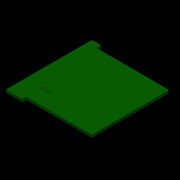
# Autodesk Inventor part: hw_DAA - PCB FPGA
Saved by Autodesk Inventor 2018 (Build 220112000, 112)
## iProperties
Created: 2024-03-13
Part Number: hw_DAA - PCB FPGA
Material: PCB
Document SubType Name: Modeling
Designer: cda1
Density: 4 g/cm^3
Appearance: PCB
Author: cda1
Autodesk Inventor part; units mm, degrees
(part 1 of 15)
ref_plane "YZ Plane" through (0, 0, 0) normal (1, 0, 0) x (0, 1, 0)
ref_plane "XZ Plane" through (0, 0, 0) normal (0, 1, 0) x (-1, 0, 0)
sketch "Boceto1" plane through (0, 0, 0) normal (0, 0, 1) x (1, 0, 0)
  line L0 (-26, 26) -> (26, 26)
  line L1 (26, 26) -> (26, -26)
  line L2 (26, -26) -> (-26, -26)
  line L3 (-26, -26) -> (-26, 26)
  line L4 (-26, 26) -> (26, -26) construction
  line L5 (26, 26) -> (-26, -26) construction
  point P0 (0, 0)
  dimension "d0" = 52
  dimension "d1" = 52
  constraints: 12 end point, 2 midpoint, 2 parallel, 1 horizontal, 1 perpendicular
  measures "d0" distance of L1.end L2.end
  measures "d1" distance of L0.end L1.end
extrude "Extrusión1" add sketch "Boceto1" against normal blind 1.742
fillet "Empalme1" radius 0.5 4 edges at (26, 26, -0.871) (-26, 26, -0.871) (-26, -26, -0.871) (26, -26, -0.871)
ref_plane "Plano de trabajo1" through (0, 0, -1.742) normal (0, 0, 1) x (1, 0, 0)
sketch "Boceto5" plane through (0, 0, 0) normal (0, 0, 1) x (1, 0, 0)
  arc A0 (25.5, -26) -> (26, -25.5) centre (25.5, -25.5) ccw construction
  line L0 (26, 25.5) -> (26, -25.5) construction
  arc A1 (26, 25.5) -> (25.5, 26) centre (25.5, 25.5) ccw construction
  line L1 (-25.5, 26) -> (25.5, 26) construction
  arc A2 (-25.5, 26) -> (-26, 25.5) centre (-25.5, 25.5) ccw construction
  line L2 (-26, -25.5) -> (-26, 25.5) construction
  arc A3 (-26, -25.5) -> (-25.5, -26) centre (-25.5, -25.5) ccw projected
  line L3 (25.5, -26) -> (-25.5, -26) projected
  line L4 (-26, -25.5) -> (-26, -28.5)
  line L5 (-26, -28.5) -> (-15.5, -28.5)
  line L6 (-15.5, -28.5) -> (-15.5, -26)
  point P0 (0, 0)
  dimension "d10" = 2.5
  dimension "d11" = 10.5
  constraints: 6 end point, 2 perpendicular, 1 point on line, 1 vertical
  measures "d10" distance of L5.end L6.end
  measures "d11" distance of L4.end L5.end
extrude "Extrusión3" add sketch "Boceto5" against normal up to surface (1.742 mm away)
sketch "Boceto6" plane through (0, 0, -1.742) normal (0, 0, -1) x (-1, 0, 0)
  arc A0 (-26, -25.5) -> (-25.5, -26) centre (-25.5, -25.5) ccw construction
  line L0 (-25.5, -26) -> (15.5, -26) construction
  line L1 (15.5, -28.5) -> (15.5, -26) construction
  line L2 (26, -28.5) -> (15.5, -28.5) construction
  line L3 (26, -28.5) -> (26, 25.5) construction
  arc A1 (26, 25.5) -> (25.5, 26) centre (25.5, 25.5) ccw construction
  line L4 (25.5, 26) -> (-25.5, 26) construction
  arc A2 (-25.5, 26) -> (-26, 25.5) centre (-25.5, 25.5) ccw construction
  line L5 (-26, 25.5) -> (-26, -25.5) construction
  line L6 (-26, 25.5) -> (-26, -25.5) construction
  line L7 (-26, 23) -> (20.107, 23)
  line L8 (20.107, 23) -> (20.107, 26)
  line L9 (20.107, 26) -> (-26, 26)
  line L10 (-26, 26) -> (-26, 23)
  point P0 (0, 0)
  dimension "d15" = 46.107
  dimension "d16" = 3
  constraints: 8 end point, 2 parallel, 2 point on line, 1 horizontal, 1 perpendicular
  measures "d15" distance of L9.end L8.end
  measures "d16" distance of L9.end L7.start
extrude "Extrusión4" cut sketch "Boceto6" against normal up to surface (1.742 mm away)
fillet "Empalme2" radius 1 1 edges at (26, 23, -0.871)
fillet "Empalme3" radius 0.5 5 edges at (-15.5, -28.5, -0.871) (-15.5, -26, -0.871) (-26, -28.5, -0.871) (-20.107, 23, -0.871) (-20.107, 26, -0.871)
sketch "Boceto17" plane through (0, 0, -1.742) normal (0, 0, -1) x (-1, 0, 0)
  circle A0 centre (16.175, -15.765) radius 0.37
  line L0 (26, -28) -> (26, 25.5) projected
  line L1 (25.5, -28.5) -> (16, -28.5) projected
  circle A1 centre (16.175, -17.035) radius 0.37
  circle A2 centre (14.905, -17.035) radius 0.37
  circle A3 centre (14.905, -15.765) radius 0.37
  circle A4 centre (13.635, -15.765) radius 0.37
  circle A5 centre (13.635, -17.035) radius 0.37
  circle A6 centre (12.365, -15.765) radius 0.37
  circle A7 centre (12.365, -17.035) radius 0.37
  circle A8 centre (11.095, -15.765) radius 0.37
  circle A9 centre (11.095, -17.035) radius 0.37
  circle A10 centre (9.825, -17.035) radius 0.37
  circle A11 centre (9.825, -15.765) radius 0.37
  point P0 (0, 0)
  dimension "d23" = 0.74
  dimension "d24" = 9.825
  dimension "d25" = 12.735
  dimension "d26" = 0.74
  dimension "d27" = 1.27
  dimension "d28" = 0.74
  dimension "d29" = 0.74
  dimension "d30" = 0.74
  dimension "d31" = 0.74
  dimension "d32" = 0.74
  dimension "d33" = 0.74
  dimension "d34" = 0.74
  dimension "d35" = 0.74
  dimension "d36" = 0.74
  dimension "d37" = 0.74
  dimension "d38" = 1.27
  dimension "d39" = 1.27
  dimension "d40" = 1.27
  dimension "d41" = 1.27
  dimension "d42" = 1.27
  constraints: 12 centre point, 10 horizontal alignment, 6 vertical alignment
  measures "d23" diameter of A0
  measures "d24" distance from line of L0 A0.centre
  measures "d25" distance from line of L1 A0.centre
  measures "d26" diameter of A1
  measures "d27" distance of A0.centre A1.centre
  measures "d28" diameter of A2
  measures "d29" diameter of A3
  measures "d30" diameter of A4
  measures "d31" diameter of A5
  measures "d32" diameter of A6
  measures "d33" diameter of A7
  measures "d34" diameter of A8
  measures "d35" diameter of A9
  measures "d36" diameter of A10
  measures "d37" diameter of A11
  measures "d38" distance of A1.centre A2.centre
  measures "d39" distance of A2.centre A5.centre
  measures "d40" distance of A5.centre A7.centre
  measures "d41" distance of A7.centre A9.centre
  measures "d42" distance of A9.centre A10.centre
extrude "Extrusión6" cut sketch "Boceto17" against normal up to surface (1.742 mm away)
sketch "TOP - 20240902" plane through (0, 0, 0) normal (0, 0, 1) x (1, 0, 0)
  arc A0 (-26, -28) -> (-25.5, -28.5) centre (-25.5, -28) ccw construction
  line L0 (-22.8, -32.942) -> (-22.8, -37.5)
  arc A1 (-22.8003, -37.5) -> (-22.7997, -37.5) centre (-22.8, -37.5) ccw
  arc A2 (-22.7997, -32.942) -> (-22.8003, -32.942) centre (-22.8, -32.942) ccw
  arc A3 (-23.3, -38) -> (-22.8, -37.5) centre (-23.3, -37.5) ccw
  arc A4 (-23.3, -37.9997) -> (-23.3, -38.0002) centre (-23.3, -38) ccw
  arc A5 (-22.7997, -37.5) -> (-22.8003, -37.5) centre (-22.8, -37.5) ccw
  line L1 (-23.3, -38) -> (-29.8, -38)
  arc A6 (-29.8, -37.9997) -> (-29.8, -38.0002) centre (-29.8, -38) ccw
  arc A7 (-23.3, -38.0002) -> (-23.3, -37.9997) centre (-23.3, -38) ccw
  arc A8 (-30.3, -37.5) -> (-29.8, -38) centre (-29.8, -37.5) ccw
  arc A9 (-30.2997, -37.5) -> (-30.3003, -37.5) centre (-30.3, -37.5) ccw
  arc A10 (-29.8, -38.0002) -> (-29.8, -37.9997) centre (-29.8, -38) ccw
  line L2 (-30.3, -37.5) -> (-30.3, -31.2)
  arc A11 (-30.2997, -31.2) -> (-30.3003, -31.2) centre (-30.3, -31.2) ccw
  arc A12 (-30.3003, -37.5) -> (-30.2997, -37.5) centre (-30.3, -37.5) ccw
  arc A13 (-30.3, -31.2) -> (-30.8, -30.7) centre (-30.8, -31.2) ccw
  arc A14 (-30.3003, -31.2) -> (-30.2997, -31.2) centre (-30.3, -31.2) ccw
  arc A15 (-30.8, -30.6998) -> (-30.8, -30.7002) centre (-30.8, -30.7) ccw
  line L3 (-30.8, -30.7) -> (-76.8, -30.7)
  arc A16 (-76.8, -30.6998) -> (-76.8, -30.7002) centre (-76.8, -30.7) ccw
  arc A17 (-30.8, -30.7002) -> (-30.8, -30.6998) centre (-30.8, -30.7) ccw
  arc A18 (-76.8, -30.7) -> (-77.3, -31.2) centre (-76.8, -31.2) ccw
  arc A19 (-76.8, -30.7002) -> (-76.8, -30.6998) centre (-76.8, -30.7) ccw
  arc A20 (-77.3003, -31.2) -> (-77.2998, -31.2) centre (-77.3001, -31.2) ccw
  line L4 (-77.3, -31.2) -> (-77.3, -49.2)
  arc A21 (-77.3003, -49.2) -> (-77.2998, -49.2) centre (-77.3001, -49.2) ccw
  arc A22 (-77.2998, -31.2) -> (-77.3003, -31.2) centre (-77.3001, -31.2) ccw
  arc A23 (-77.3, -49.2) -> (-75.3, -51.2) centre (-75.3, -49.2) ccw
  arc A24 (-77.2998, -49.2) -> (-77.3003, -49.2) centre (-77.3001, -49.2) ccw
  arc A25 (-75.3, -51.2002) -> (-75.3, -51.1998) centre (-75.3, -51.2) ccw
  line L5 (-75.3, -51.2) -> (-71.048, -51.2)
  arc A26 (-71.048, -51.2002) -> (-71.048, -51.1998) centre (-71.048, -51.2) ccw
  arc A27 (-75.3, -51.1998) -> (-75.3, -51.2002) centre (-75.3, -51.2) ccw
  arc A28 (-65.048, -57.2) -> (-71.048, -51.2) centre (-71.0482, -57.2002) ccw
  arc A29 (-65.0482, -57.2) -> (-65.0477, -57.2) centre (-65.048, -57.2) ccw
  arc A30 (-71.048, -51.1998) -> (-71.048, -51.2002) centre (-71.048, -51.2) ccw
  line L6 (-65.048, -57.2) -> (-65.048, -62.7)
  arc A31 (-65.0482, -62.7) -> (-65.0477, -62.7) centre (-65.048, -62.7) ccw
  arc A32 (-65.0477, -57.2) -> (-65.0482, -57.2) centre (-65.048, -57.2) ccw
  arc A33 (-65.048, -62.7) -> (-63.048, -64.7) centre (-63.048, -62.7) ccw
  arc A34 (-65.0477, -62.7) -> (-65.0482, -62.7) centre (-65.048, -62.7) ccw
  arc A35 (-63.048, -64.7002) -> (-63.048, -64.6997) centre (-63.048, -64.7) ccw
  line L7 (-63.048, -64.7) -> (-30.8, -64.7)
  arc A36 (-30.8, -64.7002) -> (-30.8, -64.6997) centre (-30.8, -64.7) ccw
  arc A37 (-63.048, -64.6997) -> (-63.048, -64.7002) centre (-63.048, -64.7) ccw
  arc A38 (-30.8, -64.7) -> (-30.3, -64.2) centre (-30.8, -64.2) ccw
  arc A39 (-30.8, -64.6997) -> (-30.8, -64.7002) centre (-30.8, -64.7) ccw
  arc A40 (-30.2997, -64.2) -> (-30.3003, -64.2) centre (-30.3, -64.2) ccw
  line L8 (-30.3, -64.2) -> (-30.3, -59.8)
  arc A41 (-30.2997, -59.8) -> (-30.3003, -59.8) centre (-30.3, -59.8) ccw
  arc A42 (-30.3003, -64.2) -> (-30.2997, -64.2) centre (-30.3, -64.2) ccw
  arc A43 (-29.8, -59.3) -> (-30.3, -59.8) centre (-29.8, -59.8) ccw
  arc A44 (-29.8, -59.3002) -> (-29.8, -59.2998) centre (-29.8, -59.3) ccw
  arc A45 (-30.3003, -59.8) -> (-30.2997, -59.8) centre (-30.3, -59.8) ccw
  line L9 (-29.8, -59.3) -> (-23.3, -59.3)
  arc A46 (-23.3, -59.3002) -> (-23.3, -59.2998) centre (-23.3, -59.3) ccw
  arc A47 (-29.8, -59.2998) -> (-29.8, -59.3002) centre (-29.8, -59.3) ccw
  arc A48 (-22.8, -59.8) -> (-23.3, -59.3) centre (-23.3, -59.8) ccw
  arc A49 (-22.8003, -59.8) -> (-22.7997, -59.8) centre (-22.8, -59.8) ccw
  arc A50 (-23.3, -59.2998) -> (-23.3, -59.3002) centre (-23.3, -59.3) ccw
  line L10 (-22.8, -59.8) -> (-22.8, -62.458)
  arc A51 (-22.8003, -62.458) -> (-22.7997, -62.458) centre (-22.8, -62.458) ccw
  arc A52 (-22.7997, -59.8) -> (-22.8003, -59.8) centre (-22.8, -59.8) ccw
  arc A53 (-22.8, -62.458) -> (-22.3, -62.958) centre (-22.3, -62.458) ccw
  arc A54 (-22.7997, -62.458) -> (-22.8003, -62.458) centre (-22.8, -62.458) ccw
  arc A55 (-22.3, -62.9582) -> (-22.3, -62.9577) centre (-22.3, -62.958) ccw
  line L11 (-22.3, -62.958) -> (-16, -62.958)
  arc A56 (-16, -62.9582) -> (-16, -62.9577) centre (-16, -62.958) ccw
  arc A57 (-22.3, -62.9577) -> (-22.3, -62.9582) centre (-22.3, -62.958) ccw
  arc A58 (-16, -62.958) -> (-15.5, -62.458) centre (-16, -62.458) ccw
  arc A59 (-16, -62.9577) -> (-16, -62.9582) centre (-16, -62.958) ccw
  arc A60 (-15.4998, -62.458) -> (-15.5002, -62.458) centre (-15.5, -62.458) ccw
  line L12 (-15.5, -62.458) -> (-15.5, -60.4)
  arc A61 (-15.4998, -60.4) -> (-15.5002, -60.4) centre (-15.5, -60.4) ccw
  arc A62 (-15.5002, -62.458) -> (-15.4998, -62.458) centre (-15.5, -62.458) ccw
  arc A63 (25.5, -120.6) -> (26, -120.1) centre (25.5, -120.1) ccw
  arc A64 (25.5, -120.5998) -> (25.5, -120.6003) centre (25.5, -120.6001) ccw
  arc A65 (26.0003, -120.1) -> (25.9998, -120.1) centre (26, -120.1) ccw
  line L13 (25.5, -120.6) -> (-25.5, -120.6)
  arc A66 (-25.5, -120.5998) -> (-25.5, -120.6003) centre (-25.5, -120.6001) ccw
  arc A67 (25.5, -120.6003) -> (25.5, -120.5998) centre (25.5, -120.6001) ccw
  arc A68 (-26, -120.1) -> (-25.5, -120.6) centre (-25.5, -120.1) ccw
  arc A69 (-25.9997, -120.1) -> (-26.0002, -120.1) centre (-26, -120.1) ccw
  arc A70 (-25.5, -120.6003) -> (-25.5, -120.5998) centre (-25.5, -120.6001) ccw
  line L14 (-26, -120.1) -> (-26, -66.6)
  arc A71 (-25.9997, -66.6) -> (-26.0002, -66.6) centre (-26, -66.6) ccw
  arc A72 (-26.0002, -120.1) -> (-25.9997, -120.1) centre (-26, -120.1) ccw
  arc A73 (-25.5, -66.1) -> (-26, -66.6) centre (-25.5, -66.6) ccw
  arc A74 (-25.5, -66.1003) -> (-25.5, -66.0997) centre (-25.5, -66.1) ccw
  arc A75 (-26.0002, -66.6) -> (-25.9997, -66.6) centre (-26, -66.6) ccw
  line L15 (-25.5, -66.1) -> (-16, -66.1)
  arc A76 (-16, -66.1003) -> (-16, -66.0997) centre (-16, -66.1) ccw
  arc A77 (-25.5, -66.0997) -> (-25.5, -66.1003) centre (-25.5, -66.1) ccw
  arc A78 (-15.5, -66.6) -> (-16, -66.1) centre (-16, -66.6) ccw
  arc A79 (-15.5002, -66.6) -> (-15.4998, -66.6) centre (-15.5, -66.6) ccw
  arc A80 (-16, -66.0997) -> (-16, -66.1003) centre (-16, -66.1) ccw
  line L16 (-15.5, -66.6) -> (-15.5, -72.9)
  arc A81 (-15.5002, -72.9) -> (-15.4998, -72.9) centre (-15.5, -72.9) ccw
  arc A82 (-15.4998, -66.6) -> (-15.5002, -66.6) centre (-15.5, -66.6) ccw
  arc A83 (-15.5, -72.9) -> (-15, -73.4) centre (-15, -72.9) ccw
  arc A84 (-15.4998, -72.9) -> (-15.5002, -72.9) centre (-15.5, -72.9) ccw
  arc A85 (-15, -73.4002) -> (-15, -73.3997) centre (-15, -73.4) ccw
  line L17 (-15, -59.9) -> (-13.5, -59.9)
  arc A86 (-13.5, -59.9002) -> (-13.5, -59.8998) centre (-13.5, -59.9) ccw
  arc A87 (-15, -59.8998) -> (-15, -59.9002) centre (-15, -59.9) ccw
  arc A88 (-13, -60.4) -> (-13.5, -59.9) centre (-13.5, -60.4) ccw
  arc A89 (-13.0002, -60.4) -> (-12.9998, -60.4) centre (-13, -60.4) ccw
  arc A90 (-13.5, -59.8998) -> (-13.5, -59.9002) centre (-13.5, -59.9) ccw
  line L18 (-13, -60.4) -> (-13, -72.9)
  arc A91 (-13.0002, -72.9) -> (-12.9998, -72.9) centre (-13, -72.9) ccw
  arc A92 (-12.9998, -60.4) -> (-13.0002, -60.4) centre (-13, -60.4) ccw
  arc A93 (-13.5, -73.4) -> (-13, -72.9) centre (-13.5, -72.9) ccw
  arc A94 (-13.5, -73.3997) -> (-13.5, -73.4002) centre (-13.5, -73.4) ccw
  arc A95 (-12.9998, -72.9) -> (-13.0002, -72.9) centre (-13, -72.9) ccw
  line L19 (-13.5, -73.4) -> (-15, -73.4)
  arc A96 (-15, -73.3997) -> (-15, -73.4002) centre (-15, -73.4) ccw
  arc A97 (-13.5, -73.4002) -> (-13.5, -73.3997) centre (-13.5, -73.4) ccw
  arc A98 (26, -73.9) -> (25.5, -73.4) centre (25.5, -73.9) ccw
  arc A99 (25.9998, -73.9) -> (26.0003, -73.9) centre (26, -73.9) ccw
  arc A100 (25.5, -73.3997) -> (25.5, -73.4002) centre (25.5, -73.4) ccw
  line L20 (26, -73.9) -> (26, -120.1)
  arc A101 (25.9998, -120.1) -> (26.0003, -120.1) centre (26, -120.1) ccw
  arc A102 (26.0003, -73.9) -> (25.9998, -73.9) centre (26, -73.9) ccw
  line L21 (7.4, 23.5) -> (7.4, 31.9)
  arc A103 (7.4002, 31.9) -> (7.3998, 31.9) centre (7.4, 31.9) ccw
  arc A104 (7.3998, 23.5) -> (7.4002, 23.5) centre (7.4, 23.5) ccw
  arc A105 (7.9, 32.4) -> (7.4, 31.9) centre (7.9, 31.9) ccw
  arc A106 (7.9, 32.3998) -> (7.9, 32.4002) centre (7.9, 32.4) ccw
  arc A107 (7.3998, 31.9) -> (7.4002, 31.9) centre (7.4, 31.9) ccw
  line L22 (7.9, 32.4) -> (12.55, 32.4)
  arc A108 (12.55, 32.3998) -> (12.55, 32.4002) centre (12.55, 32.4) ccw
  arc A109 (7.9, 32.4002) -> (7.9, 32.3998) centre (7.9, 32.4) ccw
  arc A110 (7.4, 23.5) -> (7.9, 23) centre (7.9, 23.5) ccw
  arc A111 (7.4002, 23.5) -> (7.3998, 23.5) centre (7.4, 23.5) ccw
  arc A112 (7.9, 22.9998) -> (7.9, 23.0002) centre (7.9, 23) ccw
  line L23 (7.9, 23) -> (25, 23)
  arc A113 (25, 22.9998) -> (25, 23.0002) centre (25, 23) ccw
  arc A114 (7.9, 23.0002) -> (7.9, 22.9998) centre (7.9, 23) ccw
  arc A115 (12.55, 32.4) -> (13.05, 32.9) centre (12.55, 32.9) ccw
  arc A116 (12.55, 32.4002) -> (12.55, 32.3998) centre (12.55, 32.4) ccw
  arc A117 (13.0503, 32.9) -> (13.0498, 32.9) centre (13.05, 32.9) ccw
  line L24 (13.05, 32.9) -> (13.05, 40.1)
  arc A118 (13.0503, 40.1) -> (13.0498, 40.1) centre (13.05, 40.1) ccw
  arc A119 (13.0498, 32.9) -> (13.0503, 32.9) centre (13.05, 32.9) ccw
  arc A120 (13.55, 40.6) -> (13.05, 40.1) centre (13.55, 40.1) ccw
  arc A121 (13.55, 40.5998) -> (13.55, 40.6003) centre (13.55, 40.6) ccw
  arc A122 (13.0498, 40.1) -> (13.0503, 40.1) centre (13.05, 40.1) ccw
  line L25 (13.55, 40.6) -> (36.8, 40.6)
  arc A123 (36.8, 40.5998) -> (36.8, 40.6003) centre (36.8, 40.6) ccw
  arc A124 (13.55, 40.6003) -> (13.55, 40.5998) centre (13.55, 40.6) ccw
  arc A125 (37.3, 40.1) -> (36.8, 40.6) centre (36.8, 40.1) ccw
  arc A126 (37.2998, 40.1) -> (37.3003, 40.1) centre (37.3, 40.1) ccw
  arc A127 (36.8, 40.6003) -> (36.8, 40.5998) centre (36.8, 40.6) ccw
  line L26 (37.3, 40.1) -> (37.3, 36)
  arc A128 (37.2998, 36) -> (37.3003, 36) centre (37.3, 36) ccw
  arc A129 (37.3003, 40.1) -> (37.2998, 40.1) centre (37.3, 40.1) ccw
  arc A130 (36.8, 35.5) -> (37.3, 36) centre (36.8, 36) ccw
  arc A131 (36.8, 35.5002) -> (36.8, 35.4998) centre (36.8, 35.5) ccw
  arc A132 (37.3003, 36) -> (37.2998, 36) centre (37.3, 36) ccw
  line L27 (36.8, 35.5) -> (34.4, 35.5)
  arc A133 (34.4, 35.5002) -> (34.4, 35.4998) centre (34.4, 35.5) ccw
  arc A134 (36.8, 35.4998) -> (36.8, 35.5002) centre (36.8, 35.5) ccw
  arc A135 (34.4, 35.5) -> (33.9, 35) centre (34.4, 35) ccw
  arc A136 (34.4, 35.4998) -> (34.4, 35.5002) centre (34.4, 35.5) ccw
  arc A137 (33.8998, 35) -> (33.9002, 35) centre (33.9, 35) ccw
  line L28 (33.9, 35) -> (33.9, 30.9)
  arc A138 (33.8998, 30.9) -> (33.9002, 30.9) centre (33.9, 30.9) ccw
  arc A139 (33.9002, 35) -> (33.8998, 35) centre (33.9, 35) ccw
  arc A140 (33.9, 30.9) -> (34.4, 30.4) centre (34.4, 30.9) ccw
  arc A141 (33.9002, 30.9) -> (33.8998, 30.9) centre (33.9, 30.9) ccw
  arc A142 (34.4, 30.3998) -> (34.4, 30.4002) centre (34.4, 30.4) ccw
  line L29 (38.9, 31.8) -> (38.9, 30.9)
  arc A143 (38.8998, 30.9) -> (38.9002, 30.9) centre (38.9, 30.9) ccw
  arc A144 (38.9002, 31.8) -> (38.8998, 31.8) centre (38.9, 31.8) ccw
  arc A145 (38.4, 30.4) -> (38.9, 30.9) centre (38.4, 30.9) ccw
  arc A146 (38.4, 30.4002) -> (38.4, 30.3998) centre (38.4, 30.4) ccw
  arc A147 (38.9002, 30.9) -> (38.8998, 30.9) centre (38.9, 30.9) ccw
  line L30 (38.4, 30.4) -> (34.4, 30.4)
  arc A148 (34.4, 30.4002) -> (34.4, 30.3998) centre (34.4, 30.4) ccw
  arc A149 (38.4, 30.3998) -> (38.4, 30.4002) centre (38.4, 30.4) ccw
  line L31 (77.3, 32.8) -> (77.3, 50.2)
  arc A150 (77.3002, 50.2) -> (77.2998, 50.2) centre (77.3, 50.2) ccw
  arc A151 (77.2998, 32.8) -> (77.3002, 32.8) centre (77.3, 32.8) ccw
  arc A152 (77.8, 50.7) -> (77.3, 50.2) centre (77.8, 50.2) ccw
  arc A153 (77.8, 50.6998) -> (77.8, 50.7003) centre (77.8, 50.7) ccw
  arc A154 (77.2998, 50.2) -> (77.3002, 50.2) centre (77.3, 50.2) ccw
  line L32 (77.8, 50.7) -> (79.8, 50.7)
  arc A155 (79.8, 50.6998) -> (79.8, 50.7003) centre (79.8, 50.7) ccw
  arc A156 (77.8, 50.7003) -> (77.8, 50.6998) centre (77.8, 50.7) ccw
  arc A157 (79.8, 50.7) -> (80.3, 51.2) centre (79.8, 51.2) ccw
  arc A158 (79.8, 50.7003) -> (79.8, 50.6998) centre (79.8, 50.7) ccw
  arc A159 (80.3002, 51.2) -> (80.2998, 51.2) centre (80.3, 51.2) ccw
  line L33 (80.3, 51.2) -> (80.3, 56.4)
  arc A160 (80.3002, 56.4) -> (80.2998, 56.4) centre (80.3, 56.4) ccw
  arc A161 (80.2998, 51.2) -> (80.3002, 51.2) centre (80.3, 51.2) ccw
  arc A162 (80.3, 56.4) -> (79.8, 56.9) centre (79.8, 56.4) ccw
  arc A163 (80.2998, 56.4) -> (80.3002, 56.4) centre (80.3, 56.4) ccw
  arc A164 (79.8, 56.9002) -> (79.8, 56.8998) centre (79.8, 56.9) ccw
  line L34 (79.8, 56.9) -> (58.9, 56.9)
  arc A165 (58.9, 56.9002) -> (58.9, 56.8998) centre (58.9, 56.9) ccw
  arc A166 (79.8, 56.8998) -> (79.8, 56.9002) centre (79.8, 56.9) ccw
  line L35 (54.4, 31.3) -> (57.9, 31.3)
  arc A167 (57.9, 31.2998) -> (57.9, 31.3002) centre (57.9, 31.3) ccw
  arc A168 (54.4, 31.3002) -> (54.4, 31.2998) centre (54.4, 31.3) ccw
  arc A169 (57.9, 31.3) -> (58.4, 31.8) centre (57.9, 31.8) ccw
  arc A170 (57.9, 31.3002) -> (57.9, 31.2998) centre (57.9, 31.3) ccw
  arc A171 (58.4003, 31.8) -> (58.3998, 31.8) centre (58.4, 31.8) ccw
  arc A172 (58.9, 32.3) -> (58.4, 31.8) centre (58.9, 31.8) ccw
  arc A173 (58.9, 32.2998) -> (58.9, 32.3002) centre (58.9, 32.3) ccw
  arc A174 (58.3998, 31.8) -> (58.4003, 31.8) centre (58.4, 31.8) ccw
  line L36 (58.9, 32.3) -> (76.8, 32.3)
  arc A175 (76.8, 32.2998) -> (76.8, 32.3002) centre (76.8, 32.3) ccw
  arc A176 (58.9, 32.3002) -> (58.9, 32.2998) centre (58.9, 32.3) ccw
  arc A177 (76.8, 32.3) -> (77.3, 32.8) centre (76.8, 32.8) ccw
  arc A178 (76.8, 32.3002) -> (76.8, 32.2998) centre (76.8, 32.3) ccw
  arc A179 (77.3002, 32.8) -> (77.2998, 32.8) centre (77.3, 32.8) ccw
  arc A180 (53.9, 31.8) -> (54.4, 31.3) centre (54.4, 31.8) ccw
  arc A181 (53.9003, 31.8) -> (53.8998, 31.8) centre (53.9, 31.8) ccw
  arc A182 (54.4, 31.2998) -> (54.4, 31.3002) centre (54.4, 31.3) ccw
  arc A183 (53.9, 31.8) -> (53.4, 32.3) centre (53.4, 31.8) ccw
  arc A184 (53.8998, 31.8) -> (53.9003, 31.8) centre (53.9, 31.8) ccw
  arc A185 (53.4, 32.3002) -> (53.4, 32.2998) centre (53.4, 32.3) ccw
  line L37 (53.4, 32.3) -> (39.4, 32.3)
  arc A186 (39.4, 32.3002) -> (39.4, 32.2998) centre (39.4, 32.3) ccw
  arc A187 (53.4, 32.2998) -> (53.4, 32.3002) centre (53.4, 32.3) ccw
  arc A188 (39.4, 32.3) -> (38.9, 31.8) centre (39.4, 31.8) ccw
  arc A189 (39.4, 32.2998) -> (39.4, 32.3002) centre (39.4, 32.3) ccw
  arc A190 (38.8998, 31.8) -> (38.9002, 31.8) centre (38.9, 31.8) ccw
  line L38 (36.8, 52) -> (13.55, 52)
  arc A191 (13.55, 52.0003) -> (13.55, 51.9998) centre (13.55, 52) ccw
  arc A192 (36.8, 51.9998) -> (36.8, 52.0003) centre (36.8, 52) ccw
  arc A193 (13.05, 52.5) -> (13.55, 52) centre (13.55, 52.5) ccw
  arc A194 (13.0503, 52.5) -> (13.0498, 52.5) centre (13.05, 52.5) ccw
  arc A195 (13.55, 51.9998) -> (13.55, 52.0003) centre (13.55, 52) ccw
  line L39 (13.05, 52.5) -> (13.05, 59.358)
  arc A196 (13.0503, 59.358) -> (13.0498, 59.358) centre (13.05, 59.358) ccw
  arc A197 (13.0498, 52.5) -> (13.0503, 52.5) centre (13.05, 52.5) ccw
  arc A198 (13.05, 59.358) -> (12.55, 59.858) centre (12.55, 59.358) ccw
  arc A199 (13.0498, 59.358) -> (13.0503, 59.358) centre (13.05, 59.358) ccw
  arc A200 (12.55, 59.8582) -> (12.55, 59.8578) centre (12.55, 59.858) ccw
  line L40 (12.55, 59.858) -> (-27.242, 59.858)
  arc A201 (-27.242, 59.8582) -> (-27.242, 59.8578) centre (-27.242, 59.858) ccw
  arc A202 (12.55, 59.8578) -> (12.55, 59.8582) centre (12.55, 59.858) ccw
  arc A203 (36.8, 52) -> (37.3, 52.5) centre (36.8, 52.5) ccw
  arc A204 (36.8, 52.0003) -> (36.8, 51.9998) centre (36.8, 52) ccw
  arc A205 (37.3003, 52.5) -> (37.2998, 52.5) centre (37.3, 52.5) ccw
  line L41 (37.3, 52.5) -> (37.3, 53.2)
  arc A206 (37.3003, 53.2) -> (37.2998, 53.2) centre (37.3, 53.2) ccw
  arc A207 (37.2998, 52.5) -> (37.3003, 52.5) centre (37.3, 52.5) ccw
  arc A208 (-27.242, 59.858) -> (-27.742, 59.358) centre (-27.242, 59.358) ccw
  arc A209 (-27.242, 59.8578) -> (-27.242, 59.8582) centre (-27.242, 59.858) ccw
  arc A210 (-27.7423, 59.358) -> (-27.7417, 59.358) centre (-27.742, 59.358) ccw
  line L42 (-27.742, 59.358) -> (-27.742, 29.842)
  arc A211 (-27.7423, 29.842) -> (-27.7417, 29.842) centre (-27.742, 29.842) ccw
  arc A212 (-27.7417, 59.358) -> (-27.7423, 59.358) centre (-27.742, 59.358) ccw
  arc A213 (37.3, 53.2) -> (36.8, 53.7) centre (36.8, 53.2) ccw
  arc A214 (37.2998, 53.2) -> (37.3003, 53.2) centre (37.3, 53.2) ccw
  arc A215 (36.8, 53.7003) -> (36.8, 53.6998) centre (36.8, 53.7) ccw
  line L43 (36.8, 53.7) -> (34.4, 53.7)
  arc A216 (34.4, 53.7003) -> (34.4, 53.6998) centre (34.4, 53.7) ccw
  arc A217 (36.8, 53.6998) -> (36.8, 53.7003) centre (36.8, 53.7) ccw
  arc A218 (33.9, 54.2) -> (34.4, 53.7) centre (34.4, 54.2) ccw
  arc A219 (33.9002, 54.2) -> (33.8998, 54.2) centre (33.9, 54.2) ccw
  arc A220 (34.4, 53.6998) -> (34.4, 53.7003) centre (34.4, 53.7) ccw
  line L44 (33.9, 54.2) -> (33.9, 58.3)
  arc A221 (33.9002, 58.3) -> (33.8998, 58.3) centre (33.9, 58.3) ccw
  arc A222 (33.8998, 54.2) -> (33.9002, 54.2) centre (33.9, 54.2) ccw
  line L45 (-15, -26) -> (-13.5, -26)
  arc A223 (-13.5, -26.0002) -> (-13.5, -25.9997) centre (-13.5, -26) ccw
  arc A224 (-15, -25.9997) -> (-15, -26.0002) centre (-15, -26) ccw
  arc A225 (-13, -26.5) -> (-13.5, -26) centre (-13.5, -26.5) ccw
  arc A226 (-13.0002, -26.5) -> (-12.9998, -26.5) centre (-13, -26.5) ccw
  arc A227 (-13.5, -25.9997) -> (-13.5, -26.0002) centre (-13.5, -26) ccw
  line L46 (-13, -26.5) -> (-13, -35)
  arc A228 (-13.0002, -35) -> (-12.9998, -35) centre (-13, -35) ccw
  arc A229 (-12.9998, -26.5) -> (-13.0002, -26.5) centre (-13, -26.5) ccw
  arc A230 (-13.5, -35.5) -> (-13, -35) centre (-13.5, -35) ccw
  arc A231 (-13.5, -35.4997) -> (-13.5, -35.5002) centre (-13.5, -35.5) ccw
  arc A232 (-12.9998, -35) -> (-13.0002, -35) centre (-13, -35) ccw
  line L47 (-13.5, -35.5) -> (-15, -35.5)
  arc A233 (-15, -35.4997) -> (-15, -35.5002) centre (-15, -35.5) ccw
  arc A234 (-13.5, -35.5002) -> (-13.5, -35.4997) centre (-13.5, -35.5) ccw
  arc A235 (-15, -26) -> (-15.5, -26.5) centre (-15, -26.5) ccw
  arc A236 (-15, -26.0002) -> (-15, -25.9997) centre (-15, -26) ccw
  arc A237 (-15.5002, -26.5) -> (-15.4998, -26.5) centre (-15.5, -26.5) ccw
  line L48 (-15.5, -26.5) -> (-15.5, -28)
  arc A238 (-15.5002, -28) -> (-15.4998, -28) centre (-15.5, -28) ccw
  arc A239 (-15.4998, -26.5) -> (-15.5002, -26.5) centre (-15.5, -26.5) ccw
  arc A240 (-16, -28.5) -> (-15.5, -28) centre (-16, -28) ccw
  arc A241 (-16, -28.4997) -> (-16, -28.5002) centre (-16, -28.5) ccw
  arc A242 (-15.4998, -28) -> (-15.5002, -28) centre (-15.5, -28) ccw
  line L49 (-16, -28.5) -> (-25.5, -28.5)
  arc A243 (-25.5, -28.4997) -> (-25.5, -28.5002) centre (-25.5, -28.5) ccw
  arc A244 (-16, -28.5002) -> (-16, -28.4997) centre (-16, -28.5) ccw
  arc A245 (-26, -28) -> (-25.5, -28.5) centre (-25.5, -28) ccw
  arc A246 (-25.9997, -28) -> (-26.0002, -28) centre (-26, -28) ccw
  arc A247 (-25.5, -28.5002) -> (-25.5, -28.4997) centre (-25.5, -28.5) ccw
  line L50 (-26, -28) -> (-26, 25.5)
  arc A248 (-25.9997, 25.5) -> (-26.0002, 25.5) centre (-26, 25.5) ccw
  arc A249 (-26.0002, -28) -> (-25.9997, -28) centre (-26, -28) ccw
  arc A250 (-25.5, 26) -> (-26, 25.5) centre (-25.5, 25.5) ccw
  arc A251 (-25.5, 25.9998) -> (-25.5, 26.0002) centre (-25.5, 26) ccw
  arc A252 (-26.0002, 25.5) -> (-25.9997, 25.5) centre (-26, 25.5) ccw
  line L51 (-25.5, 26) -> (-20.6, 26)
  arc A253 (-20.6, 25.9998) -> (-20.6, 26.0002) centre (-20.6, 26) ccw
  arc A254 (-25.5, 26.0002) -> (-25.5, 25.9998) centre (-25.5, 26) ccw
  arc A255 (-20.1, 25.5) -> (-20.6, 26) centre (-20.6, 25.5) ccw
  arc A256 (-20.1002, 25.5) -> (-20.0998, 25.5) centre (-20.1, 25.5) ccw
  arc A257 (-20.6, 26.0002) -> (-20.6, 25.9998) centre (-20.6, 26) ccw
  line L52 (-20.1, 25.5) -> (-20.1, 23.5)
  arc A258 (-20.1002, 23.5) -> (-20.0998, 23.5) centre (-20.1, 23.5) ccw
  arc A259 (-20.0998, 25.5) -> (-20.1002, 25.5) centre (-20.1, 25.5) ccw
  arc A260 (-20.1, 23.5) -> (-19.6, 23) centre (-19.6, 23.5) ccw
  arc A261 (-20.0998, 23.5) -> (-20.1002, 23.5) centre (-20.1, 23.5) ccw
  arc A262 (-19.6, 22.9998) -> (-19.6, 23.0002) centre (-19.6, 23) ccw
  line L53 (-19.6, 32.4) -> (-18.3, 32.4)
  arc A263 (-18.3, 32.3998) -> (-18.3, 32.4002) centre (-18.3, 32.4) ccw
  arc A264 (-19.6, 32.4002) -> (-19.6, 32.3998) centre (-19.6, 32.4) ccw
  arc A265 (-17.8, 31.9) -> (-18.3, 32.4) centre (-18.3, 31.9) ccw
  arc A266 (-17.8002, 31.9) -> (-17.7998, 31.9) centre (-17.8, 31.9) ccw
  arc A267 (-18.3, 32.4002) -> (-18.3, 32.3998) centre (-18.3, 32.4) ccw
  line L54 (-17.8, 31.9) -> (-17.8, 23.5)
  arc A268 (-17.8002, 23.5) -> (-17.7998, 23.5) centre (-17.8, 23.5) ccw
  arc A269 (-17.7998, 31.9) -> (-17.8002, 31.9) centre (-17.8, 31.9) ccw
  arc A270 (-18.3, 23) -> (-17.8, 23.5) centre (-18.3, 23.5) ccw
  arc A271 (-18.3, 23.0002) -> (-18.3, 22.9998) centre (-18.3, 23) ccw
  arc A272 (-17.7998, 23.5) -> (-17.8002, 23.5) centre (-17.8, 23.5) ccw
  line L55 (-18.3, 23) -> (-19.6, 23)
  arc A273 (-19.6, 23.0002) -> (-19.6, 22.9998) centre (-19.6, 23) ccw
  arc A274 (-18.3, 22.9998) -> (-18.3, 23.0002) centre (-18.3, 23) ccw
  arc A275 (26, 22) -> (25, 23) centre (25, 22) ccw
  arc A276 (25.9998, 22) -> (26.0003, 22) centre (26, 22) ccw
  arc A277 (25, 23.0002) -> (25, 22.9998) centre (25, 23) ccw
  line L56 (26, 22) -> (26, -25.5)
  arc A278 (25.9998, -25.5) -> (26.0003, -25.5) centre (26, -25.5) ccw
  arc A279 (26.0003, 22) -> (25.9998, 22) centre (26, 22) ccw
  arc A280 (25.5, -26) -> (26, -25.5) centre (25.5, -25.5) ccw
  arc A281 (25.5, -25.9997) -> (25.5, -26.0002) centre (25.5, -26) ccw
  arc A282 (26.0003, -25.5) -> (25.9998, -25.5) centre (26, -25.5) ccw
  line L57 (-15.5, -35) -> (-15.5, -32.942)
  arc A283 (-15.4998, -32.942) -> (-15.5002, -32.942) centre (-15.5, -32.942) ccw
  arc A284 (-15.5002, -35) -> (-15.4998, -35) centre (-15.5, -35) ccw
  arc A285 (-15.5, -32.942) -> (-16, -32.442) centre (-16, -32.942) ccw
  arc A286 (-15.5002, -32.942) -> (-15.4998, -32.942) centre (-15.5, -32.942) ccw
  arc A287 (-16, -32.4418) -> (-16, -32.4422) centre (-16, -32.442) ccw
  line L58 (-16, -32.442) -> (-22.3, -32.442)
  arc A288 (-22.3, -32.4418) -> (-22.3, -32.4422) centre (-22.3, -32.442) ccw
  arc A289 (-16, -32.4422) -> (-16, -32.4418) centre (-16, -32.442) ccw
  arc A290 (-22.3, -32.442) -> (-22.8, -32.942) centre (-22.3, -32.942) ccw
  arc A291 (-22.3, -32.4422) -> (-22.3, -32.4418) centre (-22.3, -32.442) ccw
  arc A292 (-22.8003, -32.942) -> (-22.7997, -32.942) centre (-22.8, -32.942) ccw
  arc A293 (-15, -59.9) -> (-15.5, -60.4) centre (-15, -60.4) ccw
  arc A294 (-15, -59.9002) -> (-15, -59.8998) centre (-15, -59.9) ccw
  arc A295 (-15.5002, -60.4) -> (-15.4998, -60.4) centre (-15.5, -60.4) ccw
  arc A296 (25.5, -59.9) -> (26, -59.4) centre (25.5, -59.4) ccw
  arc A297 (25.5, -59.8998) -> (25.5, -59.9002) centre (25.5, -59.9) ccw
  arc A298 (26.0003, -59.4) -> (25.9998, -59.4) centre (26, -59.4) ccw
  line L59 (26, -59.4) -> (26, -36)
  arc A299 (26.0003, -36) -> (25.9998, -36) centre (26, -36) ccw
  arc A300 (25.9998, -59.4) -> (26.0003, -59.4) centre (26, -59.4) ccw
  arc A301 (26, -36) -> (25.5, -35.5) centre (25.5, -36) ccw
  arc A302 (25.9998, -36) -> (26.0003, -36) centre (26, -36) ccw
  arc A303 (25.5, -35.4997) -> (25.5, -35.5002) centre (25.5, -35.5) ccw
  arc A304 (-15.5, -35) -> (-15, -35.5) centre (-15, -35) ccw
  arc A305 (-15.4998, -35) -> (-15.5002, -35) centre (-15.5, -35) ccw
  arc A306 (-15, -35.5002) -> (-15, -35.4997) centre (-15, -35.5) ccw
  line L60 (25.5, -73.4) -> (25, -73.4)
  arc A307 (25, -73.3997) -> (25, -73.4002) centre (25, -73.4) ccw
  arc A308 (25.5, -73.4002) -> (25.5, -73.3997) centre (25.5, -73.4) ccw
  arc A309 (24.5, -72.9) -> (25, -73.4) centre (25, -72.9) ccw
  arc A310 (24.5003, -72.9) -> (24.4998, -72.9) centre (24.5, -72.9) ccw
  arc A311 (25, -73.4002) -> (25, -73.3997) centre (25, -73.4) ccw
  line L61 (24.5, -72.9) -> (24.5, -60.4)
  arc A312 (24.5003, -60.4) -> (24.4998, -60.4) centre (24.5, -60.4) ccw
  arc A313 (24.4998, -72.9) -> (24.5003, -72.9) centre (24.5, -72.9) ccw
  arc A314 (25, -59.9) -> (24.5, -60.4) centre (25, -60.4) ccw
  arc A315 (25, -59.9002) -> (25, -59.8998) centre (25, -59.9) ccw
  arc A316 (24.4998, -60.4) -> (24.5003, -60.4) centre (24.5, -60.4) ccw
  line L62 (25, -59.9) -> (25.5, -59.9)
  arc A317 (25.5, -59.9002) -> (25.5, -59.8998) centre (25.5, -59.9) ccw
  arc A318 (25, -59.8998) -> (25, -59.9002) centre (25, -59.9) ccw
  line L63 (24.5, -35) -> (24.5, -26.5)
  arc A319 (24.5003, -26.5) -> (24.4998, -26.5) centre (24.5, -26.5) ccw
  arc A320 (24.4998, -35) -> (24.5003, -35) centre (24.5, -35) ccw
  arc A321 (25, -26) -> (24.5, -26.5) centre (25, -26.5) ccw
  arc A322 (25, -26.0002) -> (25, -25.9997) centre (25, -26) ccw
  arc A323 (24.4998, -26.5) -> (24.5003, -26.5) centre (24.5, -26.5) ccw
  line L64 (25, -26) -> (25.5, -26)
  arc A324 (25.5, -26.0002) -> (25.5, -25.9997) centre (25.5, -26) ccw
  arc A325 (25, -25.9997) -> (25, -26.0002) centre (25, -26) ccw
  arc A326 (24.5, -35) -> (25, -35.5) centre (25, -35) ccw
  arc A327 (24.5003, -35) -> (24.4998, -35) centre (24.5, -35) ccw
  arc A328 (25, -35.5002) -> (25, -35.4997) centre (25, -35.5) ccw
  line L65 (25, -35.5) -> (25.5, -35.5)
  arc A329 (25.5, -35.5002) -> (25.5, -35.4997) centre (25.5, -35.5) ccw
  arc A330 (25, -35.4997) -> (25, -35.5002) centre (25, -35.5) ccw
  arc A331 (-27.742, 29.842) -> (-27.242, 29.342) centre (-27.242, 29.842) ccw
  arc A332 (-27.7417, 29.842) -> (-27.7423, 29.842) centre (-27.742, 29.842) ccw
  arc A333 (-27.242, 29.3418) -> (-27.242, 29.3423) centre (-27.242, 29.342) ccw
  line L66 (-27.242, 29.342) -> (-20.6, 29.342)
  arc A334 (-20.6, 29.3418) -> (-20.6, 29.3423) centre (-20.6, 29.342) ccw
  arc A335 (-27.242, 29.3423) -> (-27.242, 29.3418) centre (-27.242, 29.342) ccw
  arc A336 (-20.6, 29.342) -> (-20.1, 29.842) centre (-20.6, 29.842) ccw
  arc A337 (-20.6, 29.3423) -> (-20.6, 29.3418) centre (-20.6, 29.342) ccw
  arc A338 (-20.0998, 29.842) -> (-20.1002, 29.842) centre (-20.1, 29.842) ccw
  line L67 (-20.1, 29.842) -> (-20.1, 31.9)
  arc A339 (-20.0998, 31.9) -> (-20.1002, 31.9) centre (-20.1, 31.9) ccw
  arc A340 (-20.1002, 29.842) -> (-20.0998, 29.842) centre (-20.1, 29.842) ccw
  arc A341 (-19.6, 32.4) -> (-20.1, 31.9) centre (-19.6, 31.9) ccw
  arc A342 (-19.6, 32.3998) -> (-19.6, 32.4002) centre (-19.6, 32.4) ccw
  arc A343 (-20.1002, 31.9) -> (-20.0998, 31.9) centre (-20.1, 31.9) ccw
  arc A344 (34.4, 58.8) -> (33.9, 58.3) centre (34.4, 58.3) ccw
  arc A345 (34.4, 58.7998) -> (34.4, 58.8002) centre (34.4, 58.8) ccw
  arc A346 (33.8998, 58.3) -> (33.9002, 58.3) centre (33.9, 58.3) ccw
  arc A347 (58.4, 57.4) -> (58.9, 56.9) centre (58.9, 57.4) ccw
  arc A348 (58.4003, 57.4) -> (58.3998, 57.4) centre (58.4, 57.4) ccw
  arc A349 (58.9, 56.8998) -> (58.9, 56.9002) centre (58.9, 56.9) ccw
  arc A350 (58.4, 57.4) -> (57.9, 57.9) centre (57.9, 57.4) ccw
  arc A351 (58.3998, 57.4) -> (58.4003, 57.4) centre (58.4, 57.4) ccw
  arc A352 (57.9, 57.9002) -> (57.9, 57.8998) centre (57.9, 57.9) ccw
  line L68 (57.9, 57.9) -> (54.4, 57.9)
  arc A353 (54.4, 57.9002) -> (54.4, 57.8998) centre (54.4, 57.9) ccw
  arc A354 (57.9, 57.8998) -> (57.9, 57.9002) centre (57.9, 57.9) ccw
  arc A355 (54.4, 57.9) -> (53.9, 57.4) centre (54.4, 57.4) ccw
  arc A356 (54.4, 57.8998) -> (54.4, 57.9002) centre (54.4, 57.9) ccw
  arc A357 (53.8998, 57.4) -> (53.9003, 57.4) centre (53.9, 57.4) ccw
  arc A358 (53.4, 56.9) -> (53.9, 57.4) centre (53.4, 57.4) ccw
  arc A359 (53.4, 56.9002) -> (53.4, 56.8998) centre (53.4, 56.9) ccw
  arc A360 (53.9003, 57.4) -> (53.8998, 57.4) centre (53.9, 57.4) ccw
  line L69 (53.4, 56.9) -> (39.4, 56.9)
  arc A361 (39.4, 56.9002) -> (39.4, 56.8998) centre (39.4, 56.9) ccw
  arc A362 (53.4, 56.8998) -> (53.4, 56.9002) centre (53.4, 56.9) ccw
  arc A363 (38.9, 57.4) -> (39.4, 56.9) centre (39.4, 57.4) ccw
  arc A364 (38.9002, 57.4) -> (38.8998, 57.4) centre (38.9, 57.4) ccw
  arc A365 (39.4, 56.8998) -> (39.4, 56.9002) centre (39.4, 56.9) ccw
  line L70 (38.9, 57.4) -> (38.9, 58.3)
  arc A366 (38.9002, 58.3) -> (38.8998, 58.3) centre (38.9, 58.3) ccw
  arc A367 (38.8998, 57.4) -> (38.9002, 57.4) centre (38.9, 57.4) ccw
  arc A368 (38.9, 58.3) -> (38.4, 58.8) centre (38.4, 58.3) ccw
  arc A369 (38.8998, 58.3) -> (38.9002, 58.3) centre (38.9, 58.3) ccw
  arc A370 (38.4, 58.8002) -> (38.4, 58.7998) centre (38.4, 58.8) ccw
  line L71 (38.4, 58.8) -> (34.4, 58.8)
  arc A371 (34.4, 58.8002) -> (34.4, 58.7998) centre (34.4, 58.8) ccw
  arc A372 (38.4, 58.7998) -> (38.4, 58.8002) centre (38.4, 58.8) ccw
  circle A373 centre (-36.6, -61.378) radius 2
  circle A374 centre (-36.6, -34.022) radius 2
  circle A375 centre (-19.1, -36.062) radius 2
  circle A376 centre (-23.092, 32.962) radius 2
  circle A377 centre (-9.192, 56.238) radius 2
  circle A378 centre (36.4, 56.256) radius 2
  circle A379 centre (78.021, 53.178) radius 2
  circle A380 centre (36.4, 32.98) radius 2
  circle A381 centre (56.15, 55.6) radius 2
  circle A382 centre (56.15, 33.6) radius 2
  circle A383 centre (-19.1, -59.338) radius 2
  circle A384 centre (-67.2, -34.022) radius 2
  circle A385 centre (23.035, -103.86) radius 0.37
  circle A386 centre (-13.635, -15.765) radius 0.37
  circle A387 centre (22.735, -52.24) radius 0.37
  circle A388 centre (-11.095, -17.035) radius 0.37
  circle A389 centre (44.6, 53.6) radius 1.5
  circle A390 centre (-9.825, -15.765) radius 0.37
  circle A391 centre (21.765, -107.67) radius 0.37
  circle A392 centre (21.765, -103.86) radius 0.37
  circle A393 centre (-16.175, -15.765) radius 0.37
  circle A394 centre (22.735, -47.16) radius 0.37
  circle A395 centre (21.765, -108.94) radius 0.37
  circle A396 centre (-14.905, -17.035) radius 0.37
  circle A397 centre (23.035, -106.4) radius 0.37
  circle A398 centre (21.465, -48.43) radius 0.37
  circle A399 centre (22.735, -49.7) radius 0.37
  circle A400 centre (23.035, -105.13) radius 0.37
  circle A401 centre (21.465, -50.97) radius 0.37
  circle A402 centre (44.6, 35.6) radius 1.5
  circle A403 centre (21.465, -52.24) radius 0.37
  circle A404 centre (21.765, -106.4) radius 0.37
  circle A405 centre (23.035, -108.94) radius 0.37
  circle A406 centre (-16.175, -17.035) radius 0.37
  circle A407 centre (-13.635, -17.035) radius 0.37
  circle A408 centre (21.465, -47.16) radius 0.37
  circle A409 centre (21.765, -105.13) radius 0.37
  circle A410 centre (23.035, -107.67) radius 0.37
  circle A411 centre (-11.095, -15.765) radius 0.37
  circle A412 centre (73, 35.6) radius 1.5
  circle A413 centre (-12.365, -15.765) radius 0.37
  circle A414 centre (-12.365, -17.035) radius 0.37
  circle A415 centre (-14.905, -15.765) radius 0.37
  circle A416 centre (73, 53.6) radius 1.5
  circle A417 centre (22.735, -50.97) radius 0.37
  circle A418 centre (21.465, -49.7) radius 0.37
  circle A419 centre (22.735, -48.43) radius 0.37
  circle A420 centre (-9.825, -17.035) radius 0.37
  line L72 (-26.016, 50.108) -> (-23.984, 50.108)
  line L73 (-55.4108, -59.243) -> (-60.3892, -59.243)
  arc A421 (-60.3892, -59.1922) -> (-60.3892, -59.2938) centre (-60.3892, -59.243) ccw
  arc A422 (-55.4108, -59.2938) -> (-55.4108, -59.1922) centre (-55.4108, -59.243) ccw
  line L74 (-60.3892, -59.243) -> (-60.3892, -56.957)
  arc A423 (-60.3384, -56.957) -> (-60.44, -56.957) centre (-60.3892, -56.957) ccw
  arc A424 (-60.44, -59.243) -> (-60.3384, -59.243) centre (-60.3892, -59.243) ccw
  line L75 (-60.3892, -56.957) -> (-55.4108, -56.957)
  arc A425 (-55.4108, -57.0078) -> (-55.4108, -56.9062) centre (-55.4108, -56.957) ccw
  arc A426 (-60.3892, -56.9062) -> (-60.3892, -57.0078) centre (-60.3892, -56.957) ccw
  line L76 (-55.4108, -56.957) -> (-55.4108, -59.243)
  arc A427 (-55.4616, -59.243) -> (-55.36, -59.243) centre (-55.4108, -59.243) ccw
  arc A428 (-55.36, -56.957) -> (-55.4616, -56.957) centre (-55.4108, -56.957) ccw
  arc A429 (-23.984, 50.0572) -> (-23.984, 50.1588) centre (-23.984, 50.108) ccw
  line L77 (-12.543, 46.2108) -> (-12.543, 51.1892)
  arc A430 (-12.4922, 51.1892) -> (-12.5938, 51.1892) centre (-12.543, 51.1892) ccw
  arc A431 (-12.5938, 46.2108) -> (-12.4922, 46.2108) centre (-12.543, 46.2108) ccw
  line L78 (-12.543, 51.1892) -> (-10.257, 51.1892)
  arc A432 (-10.257, 51.1384) -> (-10.257, 51.24) centre (-10.257, 51.1892) ccw
  arc A433 (-12.543, 51.24) -> (-12.543, 51.1384) centre (-12.543, 51.1892) ccw
  line L79 (-10.257, 51.1892) -> (-10.257, 46.2108)
  arc A434 (-10.3078, 46.2108) -> (-10.2062, 46.2108) centre (-10.257, 46.2108) ccw
  arc A435 (-10.2062, 51.1892) -> (-10.3078, 51.1892) centre (-10.257, 51.1892) ccw
  line L80 (-10.257, 46.2108) -> (-12.543, 46.2108)
  arc A436 (-12.543, 46.2616) -> (-12.543, 46.16) centre (-12.543, 46.2108) ccw
  arc A437 (-10.257, 46.16) -> (-10.257, 46.2616) centre (-10.257, 46.2108) ccw
  arc A438 (-26.016, 50.1588) -> (-26.016, 50.0572) centre (-26.016, 50.108) ccw
  line L81 (-13.835, 47.903) -> (-13.835, 50.697)
  arc A439 (-13.7842, 50.697) -> (-13.8858, 50.697) centre (-13.835, 50.697) ccw
  arc A440 (-13.8858, 47.903) -> (-13.7842, 47.903) centre (-13.835, 47.903) ccw
  line L82 (-13.835, 50.697) -> (-12.565, 50.697)
  arc A441 (-12.565, 50.6462) -> (-12.565, 50.7478) centre (-12.565, 50.697) ccw
  arc A442 (-13.835, 50.7478) -> (-13.835, 50.6462) centre (-13.835, 50.697) ccw
  line L83 (-12.565, 50.697) -> (-12.565, 47.903)
  arc A443 (-12.6158, 47.903) -> (-12.5142, 47.903) centre (-12.565, 47.903) ccw
  arc A444 (-12.5142, 50.697) -> (-12.6158, 50.697) centre (-12.565, 50.697) ccw
  line L84 (-12.565, 47.903) -> (-13.835, 47.903)
  arc A445 (-13.835, 47.9538) -> (-13.835, 47.8522) centre (-13.835, 47.903) ccw
  arc A446 (-12.565, 47.8522) -> (-12.565, 47.9538) centre (-12.565, 47.903) ccw
  line L85 (-23.984, 50.108) -> (-23.984, 49.092)
  line L86 (-6.692, -83.684) -> (-6.692, -85.716)
  arc A447 (-6.7428, -85.716) -> (-6.6412, -85.716) centre (-6.692, -85.716) ccw
  arc A448 (-6.6412, -83.684) -> (-6.7428, -83.684) centre (-6.692, -83.684) ccw
  line L87 (-6.692, -85.716) -> (-7.708, -85.716)
  arc A449 (-7.708, -85.6652) -> (-7.708, -85.7668) centre (-7.708, -85.716) ccw
  arc A450 (-6.692, -85.7668) -> (-6.692, -85.6652) centre (-6.692, -85.716) ccw
  line L88 (-7.708, -85.716) -> (-7.708, -83.684)
  arc A451 (-7.6572, -83.684) -> (-7.7588, -83.684) centre (-7.708, -83.684) ccw
  arc A452 (-7.7588, -85.716) -> (-7.6572, -85.716) centre (-7.708, -85.716) ccw
  line L89 (-7.708, -83.684) -> (-6.692, -83.684)
  arc A453 (-6.692, -83.7348) -> (-6.692, -83.6332) centre (-6.692, -83.684) ccw
  arc A454 (-7.708, -83.6332) -> (-7.708, -83.7348) centre (-7.708, -83.684) ccw
  arc A455 (-24.0348, 49.092) -> (-23.9332, 49.092) centre (-23.984, 49.092) ccw
  line L90 (-14.865, -87.603) -> (-14.865, -90.397)
  arc A456 (-14.9158, -90.397) -> (-14.8142, -90.397) centre (-14.865, -90.397) ccw
  arc A457 (-14.8142, -87.603) -> (-14.9158, -87.603) centre (-14.865, -87.603) ccw
  line L91 (-14.865, -90.397) -> (-16.135, -90.397)
  arc A458 (-16.135, -90.3462) -> (-16.135, -90.4478) centre (-16.135, -90.397) ccw
  arc A459 (-14.865, -90.4478) -> (-14.865, -90.3462) centre (-14.865, -90.397) ccw
  line L92 (-16.135, -90.397) -> (-16.135, -87.603)
  arc A460 (-16.0842, -87.603) -> (-16.1858, -87.603) centre (-16.135, -87.603) ccw
  arc A461 (-16.1858, -90.397) -> (-16.0842, -90.397) centre (-16.135, -90.397) ccw
  line L93 (-16.135, -87.603) -> (-14.865, -87.603)
  arc A462 (-14.865, -87.6538) -> (-14.865, -87.5522) centre (-14.865, -87.603) ccw
  arc A463 (-16.135, -87.5522) -> (-16.135, -87.6538) centre (-16.135, -87.603) ccw
  arc A464 (-23.9332, 50.108) -> (-24.0348, 50.108) centre (-23.984, 50.108) ccw
  line L94 (-13.297, -95.765) -> (-10.503, -95.765)
  arc A465 (-10.503, -95.8158) -> (-10.503, -95.7142) centre (-10.503, -95.765) ccw
  arc A466 (-13.297, -95.7142) -> (-13.297, -95.8158) centre (-13.297, -95.765) ccw
  line L95 (-10.503, -95.765) -> (-10.503, -97.035)
  arc A467 (-10.5538, -97.035) -> (-10.4522, -97.035) centre (-10.503, -97.035) ccw
  arc A468 (-10.4522, -95.765) -> (-10.5538, -95.765) centre (-10.503, -95.765) ccw
  line L96 (-10.503, -97.035) -> (-13.297, -97.035)
  arc A469 (-13.297, -96.9842) -> (-13.297, -97.0858) centre (-13.297, -97.035) ccw
  arc A470 (-10.503, -97.0858) -> (-10.503, -96.9842) centre (-10.503, -97.035) ccw
  line L97 (-13.297, -97.035) -> (-13.297, -95.765)
  arc A471 (-13.2462, -95.765) -> (-13.3478, -95.765) centre (-13.297, -95.765) ccw
  arc A472 (-13.3478, -97.035) -> (-13.2462, -97.035) centre (-13.297, -97.035) ccw
  line L98 (-23.984, 49.092) -> (-26.016, 49.092)
  line L99 (-16.284, -100.108) -> (-18.316, -100.108)
  arc A473 (-18.316, -100.0572) -> (-18.316, -100.1588) centre (-18.316, -100.108) ccw
  arc A474 (-16.284, -100.1588) -> (-16.284, -100.0572) centre (-16.284, -100.108) ccw
  line L100 (-18.316, -100.108) -> (-18.316, -99.092)
  arc A475 (-18.2652, -99.092) -> (-18.3668, -99.092) centre (-18.316, -99.092) ccw
  arc A476 (-18.3668, -100.108) -> (-18.2652, -100.108) centre (-18.316, -100.108) ccw
  line L101 (-18.316, -99.092) -> (-16.284, -99.092)
  arc A477 (-16.284, -99.1428) -> (-16.284, -99.0412) centre (-16.284, -99.092) ccw
  arc A478 (-18.316, -99.0412) -> (-18.316, -99.1428) centre (-18.316, -99.092) ccw
  line L102 (-16.284, -99.092) -> (-16.284, -100.108)
  arc A479 (-16.3348, -100.108) -> (-16.2332, -100.108) centre (-16.284, -100.108) ccw
  arc A480 (-16.2332, -99.092) -> (-16.3348, -99.092) centre (-16.284, -99.092) ccw
  arc A481 (-26.016, 49.1428) -> (-26.016, 49.0412) centre (-26.016, 49.092) ccw
  line L103 (-18.308, -105.116) -> (-18.308, -103.084)
  arc A482 (-18.2572, -103.084) -> (-18.3588, -103.084) centre (-18.308, -103.084) ccw
  arc A483 (-18.3588, -105.116) -> (-18.2572, -105.116) centre (-18.308, -105.116) ccw
  line L104 (-18.308, -103.084) -> (-17.292, -103.084)
  arc A484 (-17.292, -103.1348) -> (-17.292, -103.0332) centre (-17.292, -103.084) ccw
  arc A485 (-18.308, -103.0332) -> (-18.308, -103.1348) centre (-18.308, -103.084) ccw
  line L105 (-17.292, -103.084) -> (-17.292, -105.116)
  arc A486 (-17.3428, -105.116) -> (-17.2412, -105.116) centre (-17.292, -105.116) ccw
  arc A487 (-17.2412, -103.084) -> (-17.3428, -103.084) centre (-17.292, -103.084) ccw
  line L106 (-17.292, -105.116) -> (-18.308, -105.116)
  arc A488 (-18.308, -105.0652) -> (-18.308, -105.1668) centre (-18.308, -105.116) ccw
  arc A489 (-17.292, -105.1668) -> (-17.292, -105.0652) centre (-17.292, -105.116) ccw
  arc A490 (-23.984, 49.0412) -> (-23.984, 49.1428) centre (-23.984, 49.092) ccw
  line L107 (-16.284, -101.108) -> (-18.316, -101.108)
  arc A491 (-18.316, -101.0572) -> (-18.316, -101.1588) centre (-18.316, -101.108) ccw
  arc A492 (-16.284, -101.1588) -> (-16.284, -101.0572) centre (-16.284, -101.108) ccw
  line L108 (-18.316, -101.108) -> (-18.316, -100.092)
  arc A493 (-18.2652, -100.092) -> (-18.3668, -100.092) centre (-18.316, -100.092) ccw
  arc A494 (-18.3668, -101.108) -> (-18.2652, -101.108) centre (-18.316, -101.108) ccw
  line L109 (-18.316, -100.092) -> (-16.284, -100.092)
  arc A495 (-16.284, -100.1428) -> (-16.284, -100.0412) centre (-16.284, -100.092) ccw
  arc A496 (-18.316, -100.0412) -> (-18.316, -100.1428) centre (-18.316, -100.092) ccw
  line L110 (-16.284, -100.092) -> (-16.284, -101.108)
  arc A497 (-16.3348, -101.108) -> (-16.2332, -101.108) centre (-16.284, -101.108) ccw
  arc A498 (-16.2332, -100.092) -> (-16.3348, -100.092) centre (-16.284, -100.092) ccw
  line L111 (-26.016, 49.092) -> (-26.016, 50.108)
  line L112 (-16.284, -102.108) -> (-18.316, -102.108)
  arc A499 (-18.316, -102.0572) -> (-18.316, -102.1588) centre (-18.316, -102.108) ccw
  arc A500 (-16.284, -102.1588) -> (-16.284, -102.0572) centre (-16.284, -102.108) ccw
  line L113 (-18.316, -102.108) -> (-18.316, -101.092)
  arc A501 (-18.2652, -101.092) -> (-18.3668, -101.092) centre (-18.316, -101.092) ccw
  arc A502 (-18.3668, -102.108) -> (-18.2652, -102.108) centre (-18.316, -102.108) ccw
  line L114 (-18.316, -101.092) -> (-16.284, -101.092)
  arc A503 (-16.284, -101.1428) -> (-16.284, -101.0412) centre (-16.284, -101.092) ccw
  arc A504 (-18.316, -101.0412) -> (-18.316, -101.1428) centre (-18.316, -101.092) ccw
  line L115 (-16.284, -101.092) -> (-16.284, -102.108)
  arc A505 (-16.3348, -102.108) -> (-16.2332, -102.108) centre (-16.284, -102.108) ccw
  arc A506 (-16.2332, -101.092) -> (-16.3348, -101.092) centre (-16.284, -101.092) ccw
  arc A507 (-25.9652, 50.108) -> (-26.0668, 50.108) centre (-26.016, 50.108) ccw
  line L116 (-9.765, -97.203) -> (-9.765, -99.997)
  arc A508 (-9.8158, -99.997) -> (-9.7142, -99.997) centre (-9.765, -99.997) ccw
  arc A509 (-9.7142, -97.203) -> (-9.8158, -97.203) centre (-9.765, -97.203) ccw
  line L117 (-9.765, -99.997) -> (-11.035, -99.997)
  arc A510 (-11.035, -99.9462) -> (-11.035, -100.0478) centre (-11.035, -99.997) ccw
  arc A511 (-9.765, -100.0478) -> (-9.765, -99.9462) centre (-9.765, -99.997) ccw
  line L118 (-11.035, -99.997) -> (-11.035, -97.203)
  arc A512 (-10.9842, -97.203) -> (-11.0858, -97.203) centre (-11.035, -97.203) ccw
  arc A513 (-11.0858, -99.997) -> (-10.9842, -99.997) centre (-11.035, -99.997) ccw
  line L119 (-11.035, -97.203) -> (-9.765, -97.203)
  arc A514 (-9.765, -97.2538) -> (-9.765, -97.1522) centre (-9.765, -97.203) ccw
  arc A515 (-11.035, -97.1522) -> (-11.035, -97.2538) centre (-11.035, -97.203) ccw
  arc A516 (-26.0668, 49.092) -> (-25.9652, 49.092) centre (-26.016, 49.092) ccw
  line L120 (-8.365, -99.903) -> (-8.365, -102.697)
  arc A517 (-8.4158, -102.697) -> (-8.3142, -102.697) centre (-8.365, -102.697) ccw
  arc A518 (-8.3142, -99.903) -> (-8.4158, -99.903) centre (-8.365, -99.903) ccw
  line L121 (-8.365, -102.697) -> (-9.635, -102.697)
  arc A519 (-9.635, -102.6462) -> (-9.635, -102.7478) centre (-9.635, -102.697) ccw
  arc A520 (-8.365, -102.7478) -> (-8.365, -102.6462) centre (-8.365, -102.697) ccw
  line L122 (-9.635, -102.697) -> (-9.635, -99.903)
  arc A521 (-9.5842, -99.903) -> (-9.6858, -99.903) centre (-9.635, -99.903) ccw
  arc A522 (-9.6858, -102.697) -> (-9.5842, -102.697) centre (-9.635, -102.697) ccw
  line L123 (-9.635, -99.903) -> (-8.365, -99.903)
  arc A523 (-8.365, -99.9538) -> (-8.365, -99.8522) centre (-8.365, -99.903) ccw
  arc A524 (-9.635, -99.8522) -> (-9.635, -99.9538) centre (-9.635, -99.903) ccw
  line L124 (-26.016, 46.108) -> (-23.984, 46.108)
  line L125 (-9.765, -99.903) -> (-9.765, -102.697)
  arc A525 (-9.8158, -102.697) -> (-9.7142, -102.697) centre (-9.765, -102.697) ccw
  arc A526 (-9.7142, -99.903) -> (-9.8158, -99.903) centre (-9.765, -99.903) ccw
  line L126 (-9.765, -102.697) -> (-11.035, -102.697)
  arc A527 (-11.035, -102.6462) -> (-11.035, -102.7478) centre (-11.035, -102.697) ccw
  arc A528 (-9.765, -102.7478) -> (-9.765, -102.6462) centre (-9.765, -102.697) ccw
  line L127 (-11.035, -102.697) -> (-11.035, -99.903)
  arc A529 (-10.9842, -99.903) -> (-11.0858, -99.903) centre (-11.035, -99.903) ccw
  arc A530 (-11.0858, -102.697) -> (-10.9842, -102.697) centre (-11.035, -102.697) ccw
  line L128 (-11.035, -99.903) -> (-9.765, -99.903)